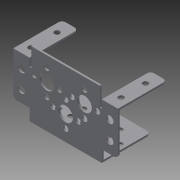
# Autodesk Inventor part: modelo 2
Saved by Autodesk Inventor 2015 (Build 190159000, 159)
## iProperties
Created: 2014-11-19
Part Number: modelo 2
Material: Generic
Document SubType Name: Modeling
Designer: alumnoutec
Density: 1 g/cm^3
Appearance: Default
Author: alumnoutec
Autodesk Inventor part; units mm, degrees
ref_plane "YZ Plane" through (0, 0, 0) normal (1, 0, 0) x (0, 1, 0)
ref_plane "XZ Plane" through (0, 0, 0) normal (0, 1, 0) x (-1, 0, 0)
ref_plane "XY Plane" through (0, 0, 0) normal (0, 0, 1) x (1, 0, 0)
sketch "Sketch2" plane through (0, 0, 0) normal (0, 1, 0) x (-1, 0, 0)
  line L0 (1.6384, 12.2587) -> (39.6384, 12.2587)
  line L1 (49.6384, 5.2687) -> (49.6384, -15.7313)
  line L2 (40.6384, -24.2313) -> (0.6384, -24.2313)
  line L3 (-8.3616, -15.7313) -> (-8.3616, 5.2687)
  line L4 (1.6384, 12.2587) -> (39.6384, 12.2587)
  line L5 (20.6384, 12.2587) -> (1.6384, 12.2587)
  line L6 (1.6384, 12.2587) -> (1.6384, 5.2687)
  line L7 (20.6384, 12.2587) -> (39.6384, 12.2587)
  line L8 (39.6384, 12.2587) -> (39.6384, 5.2687)
  circle A0 centre (31.1384, -0.7313) radius 4
  circle A1 centre (31.1384, 6.2687) radius 1.5
  circle A2 centre (24.1384, -0.7313) radius 1.5
  circle A3 centre (31.1384, -7.7313) radius 1.5
  circle A4 centre (38.1384, -0.7313) radius 1.5
  line L9 (31.1384, -0.7313) -> (40.1384, -0.7313) construction
  circle A5 centre (20.6384, -10.7313) radius 4
  circle A6 centre (20.6384, -3.7313) radius 1.5
  circle A7 centre (13.6384, -10.7313) radius 1.5
  circle A8 centre (20.6384, -17.7313) radius 1.5
  circle A9 centre (27.6384, -10.7313) radius 1.5
  line L10 (20.6384, -10.7313) -> (30.6384, -10.7313) construction
  line L11 (20.6384, 0) -> (20.6384, 3.2687)
  circle A10 centre (10.1384, -0.7313) radius 4
  circle A11 centre (10.1384, 6.2687) radius 1.5
  circle A12 centre (17.1384, -0.7313) radius 1.5
  circle A13 centre (10.1384, -7.7313) radius 1.5
  circle A14 centre (3.1384, -0.7313) radius 1.5
  line L12 (10.1384, -0.7313) -> (1.1384, -0.7313) construction
  line L13 (1.6384, 5.2687) -> (1.6384, 1.7687)
  line L14 (1.6384, 1.7687) -> (0.6384, 1.7687)
  line L15 (0.6384, 1.7687) -> (0.6384, 5.2687)
  line L16 (39.6384, 5.2687) -> (39.6384, 1.7687)
  line L17 (39.6384, 1.7687) -> (40.6384, 1.7687)
  line L18 (40.6384, 1.7687) -> (40.6384, 5.2687)
  circle A15 centre (-3.8616, -1.2313) radius 2
  circle A16 centre (-3.8616, -11.2313) radius 2
  line L19 (0.6384, 5.2687) -> (0.6384, 6.2687)
  line L20 (0.6384, 6.2687) -> (-8.3616, 6.2687)
  line L21 (-8.3616, 6.2687) -> (-8.3616, 5.2687)
  line L22 (40.6384, 5.2687) -> (40.6384, 6.2687)
  line L23 (40.6384, 6.2687) -> (49.6384, 6.2687)
  line L24 (49.6384, 6.2687) -> (49.6384, 5.2687)
  circle A17 centre (45.1384, -1.2313) radius 2
  circle A18 centre (45.1384, -11.2313) radius 2
  line L25 (0.6384, -24.2313) -> (0.6384, -17.7313)
  line L26 (0.6384, -17.7313) -> (-6.3616, -17.7313)
  line L27 (40.6384, -24.2313) -> (40.6384, -17.7313)
  line L28 (40.6384, -17.7313) -> (47.6384, -17.7313)
  arc A19 (-8.3616, -15.7313) -> (-6.3616, -17.7313) centre (-6.3616, -15.7313) ccw
  arc A20 (47.6384, -17.7313) -> (49.6384, -15.7313) centre (47.6384, -15.7313) ccw
  line L29 (1.6384, 12.2587) -> (39.6384, 12.2587)
  line L30 (40.6384, -24.2313) -> (1.6384, -24.2313)
  line L31 (1.6384, 1.7687) -> (1.6384, 12.2587)
  line L32 (40.6384, 6.2687) -> (40.6384, 1.7687)
  line L33 (40.6384, -17.7313) -> (40.6384, -24.2313)
  line L34 (49.6384, 6.2687) -> (49.6384, -15.7313)
  line L35 (-8.3616, -15.7313) -> (-8.3616, 6.2687)
  line L36 (40.6384, 6.2687) -> (49.6384, 6.2687)
  line L37 (-8.3616, 6.2687) -> (0.6384, 6.2687)
  line L38 (47.6384, -17.7313) -> (40.6384, -17.7313)
  line L39 (0.6384, -17.7313) -> (-6.3616, -17.7313)
  line L40 (-8.3616, 6.2687) -> (-8.3616, -15.7313)
  line L41 (-6.3616, -17.7313) -> (0.6384, -17.7313)
  line L42 (0.6384, -24.2313) -> (0.6384, -17.7313)
  line L43 (-6.3616, -17.7313) -> (0.6384, -17.7313)
  line L44 (0.6384, -24.2313) -> (40.6384, -24.2313)
  line L45 (40.6384, -24.2313) -> (40.6384, -17.7313)
  line L46 (40.6384, -17.7313) -> (47.6384, -17.7313)
  line L47 (49.6384, -15.7313) -> (49.6384, 6.2687)
  line L48 (49.6384, 6.2687) -> (40.6384, 6.2687)
  line L49 (40.6384, 6.2687) -> (40.6384, 1.7687)
  line L50 (39.6384, 1.7687) -> (40.6384, 1.7687)
  line L51 (39.6384, 1.7687) -> (39.6384, 12.2587)
  line L52 (39.6384, 12.2587) -> (1.6384, 12.2587)
  line L53 (1.6384, 12.2587) -> (1.6384, 1.7687)
  line L54 (1.6384, 1.7687) -> (0.6384, 1.7687)
  line L55 (0.6384, 1.7687) -> (0.6384, 6.2687)
  line L56 (0.6384, 6.2687) -> (-8.3616, 6.2687)
  line L57 (-8.3616, 6.2687) -> (-8.3616, -15.7313)
  point P0 (0, 0)
  dimension "d12" = 360
  dimension "d19" = 360
  dimension "d22" = 10
  dimension "d23" = 29
  dimension "d24" = 29
  dimension "d25" = 10.5
  dimension "d26" = 21
  dimension "d32" = 1
  dimension "d33" = 3.5
  dimension "d34" = 1
  dimension "d37" = 4
  dimension "d38" = 4
  dimension "d41" = 2
  constraints: 116 end point, 22 perpendicular, 21 centre point, 13 parallel, 10 tangent, 8 collinear, 7 symmetric about line, 6 horizontal, 5 point on circle, 3 coincident, 1 equal radius, 1 midpoint, 23 other
  measures "d22" vertical distance of A0.centre L10.start
  measures "d23" distance from line of L3 L10.start
  measures "d24" distance from line of L1 L10.start
  measures "d25" horizontal distance of A0.centre L10.start
  measures "d26" distance of A0.centre A10.centre
  measures "d32" distance of L13.end L14.end
  measures "d33" distance of L8.end L16.end
  measures "d34" distance of L16.end L17.end
  measures "d37" diameter of A15
  measures "d38" diameter of A16
  measures "d41" radius of A19
extrude "Extrusion1" add sketch "Sketch2" along normal blind 1
sketch "Sketch3" plane through (0, 1, 0) normal (0, 1, 0) x (1, 0, 0)
  line L0 (-0.6384, 17.7313) -> (-0.6384, 24.2313) projected
  line L1 (-49.6384, 15.7313) -> (-49.6384, -6.2687) projected
  line L2 (-0.6384, -1.7687) -> (-0.6384, -6.2687) projected
  line L3 (8.3616, -6.2687) -> (8.3616, 15.7313) projected
  line L4 (-40.6384, 24.2313) -> (-0.6384, 24.2313)
  line L5 (-0.6384, 24.2313) -> (-0.6384, 23.2313)
  line L6 (-0.6384, 23.2313) -> (-40.6384, 23.2313)
  line L7 (-40.6384, 23.2313) -> (-40.6384, 24.2313)
  line L8 (-0.6384, -6.2687) -> (8.3616, -6.2687)
  line L9 (8.3616, -6.2687) -> (8.3616, -5.2687)
  line L10 (8.3616, -5.2687) -> (-0.6384, -5.2687)
  line L11 (-40.6384, -6.2687) -> (-49.6384, -6.2687)
  line L12 (-49.6384, -6.2687) -> (-49.6384, -5.2687)
  line L13 (-49.6384, -5.2687) -> (-40.6384, -5.2687)
  line L14 (-40.6384, -5.2687) -> (-40.6384, -6.2687)
  line L15 (-0.6384, -5.2687) -> (-0.6384, -6.2687)
  point P0 (0, 0)
  dimension "d44" = 1
  dimension "d45" = 1
  dimension "d46" = 1
  constraints: 24 end point, 5 parallel, 5 point on line, 3 horizontal, 3 perpendicular, 1 collinear
  measures "d44" distance of L4.end L5.end
  measures "d45" distance of L9.end L8.end
  measures "d46" distance of L11.end L12.end
extrude "Extrusion2" add sketch "Sketch3" along normal blind 26
fillet "Fillet1" radius 2 6 edges at (-49.6384, 27, 5.7687) (-40.6384, 27, 5.7687) (8.3616, 27, 5.7687) (-0.6384, 27, 5.7687) (-0.6384, 27, -23.7313) (-40.6384, 27, -23.7313)
sketch "Sketch4" plane through (-40.6384, 1, -23.2313) normal (0, 0, 1) x (1, 0, 0)
  circle A0 centre (10, 12) radius 1.5
  circle A1 centre (10, 5) radius 1.5
  circle A2 centre (17, 12) radius 1.5
  circle A3 centre (10, 19) radius 1.5
  circle A4 centre (3, 12) radius 1.5
  circle A5 centre (30, 12) radius 1.5
  circle A6 centre (30, 5) radius 1.5
  circle A7 centre (37, 12) radius 1.5
  circle A8 centre (30, 19) radius 1.5
  circle A9 centre (23, 12) radius 1.5
  point P0 (40.6384, -1)
  dimension "d52" = 3
  dimension "d55" = 360
  dimension "d58" = 3
  dimension "d59" = 3
  dimension "d62" = 360
  constraints: 10 centre point, 1 coincident, 18 other
  measures "d52" diameter of A1
  measures "d58" diameter of A5
  measures "d59" diameter of A6
extrude "Extrusion3" cut sketch "Sketch4" against normal blind 26
sketch "Sketch5" plane through (-49.6384, 0, 6.2687) normal (0, 0, 1) x (1, 0, 0)
  circle A0 centre (4.5, 19.75) radius 1.5
  circle A1 centre (4.5, 5.25) radius 1.5
  line L0 (2, 27) -> (7, 27) projected
  line L1 (0, 0) -> (0, 25) projected
  line L2 (4.5, 27) -> (4.5, 12.5)
  point P0 (49.6384, 0)
  dimension "d66" = 3
  dimension "d69" = 14.5
  dimension "d70" = 7.25
  dimension "d71" = 3
  constraints: 2 centre point, 2 end point, 1 midpoint, 1 parallel
  measures "d66" diameter of A0
  measures "d69" distance of L2.start L2.end
  measures "d70" distance of A1.centre L2.end
  measures "d71" diameter of A1
extrude "Extrusion4" cut sketch "Sketch5" against normal blind 26
sketch "Sketch6" plane through (-0.6384, 0, 6.2687) normal (0, 0, 1) x (1, 0, 0)
  circle A0 centre (4.5, 19.75) radius 1.5
  circle A1 centre (4.5, 6.25) radius 1.5
  point P0 (0.6384, 0)
  dimension "d72" = 3
  dimension "d73" = 3
  constraints: 2 centre point
  measures "d72" diameter of A0
  measures "d73" diameter of A1
extrude "Extrusion5" cut sketch "Sketch6" against normal blind 26
body "Solid1"
